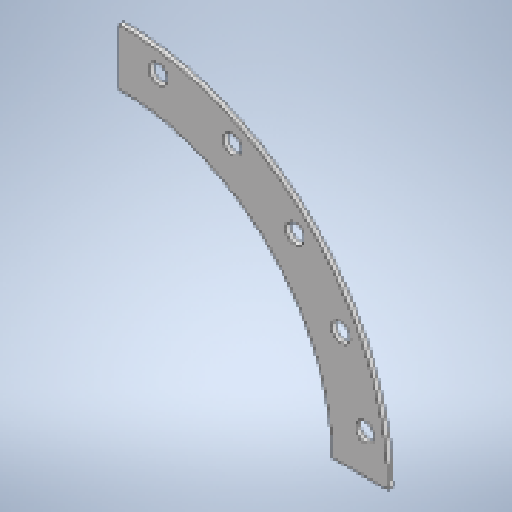
# Autodesk Inventor part: PNS-612 accses hatch flangeipt
Saved by Autodesk Inventor 2025.1 (Build 291241020, 241B)
## iProperties
Created: 2025-02-12
Part Number: PNS-612 accses hatch flangeipt
Material: Generic
Document SubType Name: Sheet Metal
Designer: pokla
Density: 1 g/cm^3
Flat Pattern Width: 33.5 cm
Flat Pattern Length: 33.5 cm
Flat Pattern Area: 1122.25 cm^2
Sheet Metal Rule: Default_mm
Sheet Metal Width: 335.000 mm
Sheet Metal Length: 335.000 mm
Sheet Metal Area: 112225.000 mm^2
Appearance: Default
Author: pokla
Autodesk Inventor part; units mm, degrees
ref_plane "YZ Plane" through (0, 0, 0) normal (1, 0, 0) x (0, 1, 0)
ref_plane "XZ Plane" through (0, 0, 0) normal (0, 1, 0) x (-1, 0, 0)
ref_plane "XY Plane" through (0, 0, 0) normal (0, 0, 1) x (1, 0, 0)
sketch "Sketch1" plane through (0, 0, 0) normal (0, 1, 0) x (-1, 0, 0)
  circle A0 centre (0, 0) radius 265
  circle A1 centre (0, 0) radius 335
  line L0 (335, 0) -> (265, 0)
  line L1 (-265, 0) -> (-335, 0)
  line L2 (0, 265) -> (0, 335)
  point P0 (300, 0)
  point P1 (-300, 0)
  point P2 (0, 300)
  dimension "d1" = 670
  dimension "d4" = 530
  constraints: 6 end point, 6 point on circle, 3 midpoint, 2 centre point, 2 coincident, 2 horizontal, 2 horizontal alignment, 1 vertical, 1 vertical alignment
  measures "d1" diameter of A1
  measures "d4" diameter of A0
extrude "Extrusion1" add sketch "Sketch1" along normal blind 6 contours A0 L1 A1 L2
sketch "Sketch2" plane through (0, 0, 0) normal (0, -1, 0) x (1, 0, 0)
  arc A0 (335, 0) -> (0, 335) centre (0, 0) ccw projected
  line L0 (0, 265) -> (0, 335) projected
  arc A1 (265, 0) -> (0, 265) centre (0, 0) ccw projected
  line L1 (335, 0) -> (265, 0) projected
  circle A2 centre (48.4947, 306.1834) radius 11.5
  arc A3 (265, 0) -> (0, 265) centre (0, 0) ccw projected
  line L2 (48.4947, 306.1834) -> (0, 0)
  dimension "d5" = 310
  dimension "d6" = 9
  dimension "d7" = 23
  constraints: 2 end point, 1 centre point
  measures "d5" distance of point (0, 0) L2.start
  measures "d6" angle of L2 L0
  measures "d7" diameter of A2
extrude "Cut1" cut sketch "Sketch2" against normal blind 8 contours A2
pattern_circular "Circular Pattern1" count 20 over 360 about axis through (0, 0, 0) along (0, 1, 0) of "Cut1"
equation "\"d4\" = Accsess_hatch_diameter"
equation "\"d9\" = Thickness"
equation "\"BendRadius\" = Thickness"
equation "\"BendReliefWidth\" = Thickness"
equation "\"BendReliefDepth\" = 0.5 * Thickness"
equation "\"CornerReliefSize\" = 4 * Thickness"
equation "\"MinimumRemnant\" = 2 * Thickness"
equation "\"TransitionRadius\" = BendRadius"
equation "\"JacobiRadiusSize\" = BendRadius"
equation "\"GapSize\" = Thickness"
equation "\"d8\" = Thickness"
equation "\"Accsess_hatch_diameter\" = 530"
equation "\"Thickness\" = 8"
body "Solid1"
